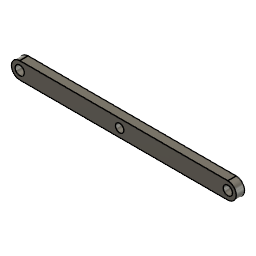
barra_direccion_v3 (Autodesk Fusion 360 design; units mm, degrees)
part number: 2026-03-15-19-52-01-353
Autodesk Fusion 360 part; units mm, degrees
sketch "Boceto1" plane through (0, 0, 0) normal (0, 0, 1) x (1, 0, 0)
  line L0 (0, -23.8223) -> (0, 23.8223) construction
  circle A0 centre (64.256, 0) radius 2.75
  line L1 (-59.344, 5) -> (64.256, 5)
  line L2 (0, 0) -> (11, 0) construction
  line L3 (-59.344, -5) -> (64.256, -5)
  arc A1 (64.256, -5) -> (64.256, 5) centre (64.256, 0) ccw
  circle A2 centre (-59.344, 0) radius 2.75
  arc A3 (-59.344, 5) -> (-59.344, -5) centre (-59.344, 0) ccw
  dimension "d1" = 5.5
  dimension "d2" = 64.256
  dimension "d4" = 10
  dimension "d10" = 5.5
  dimension "d11" = 123.6
  dimension "d12" = 5
  constraint midpoint L0 L2.start
  constraint coincident L2.start origin
  constraint vertical L0
  constraint concentric A0 A1
  constraint tangent L1 A1
  constraint horizontal L1
  constraint perpendicular L0 L2
  constraint symmetric L1.end L2 L3.end
  constraint concentric A2 A3
  constraint tangent L1 A3
  measures "d1" diameter of A0
  measures "d2" distance of L2.start A0.centre
  measures "d4" diameter of A1
  measures "d10" diameter of A2
  measures "d11" distance of A0.centre A2.centre
  measures "d12" distance of L3 A2.centre
extrude "Extruir1" add sketch "Boceto1" along normal blind 5
sketch "Boceto2" plane through (0, 0, 5) normal (0, 0, 1) x (1, 0, 0)
  circle A0 centre (64.256, 0) radius 2.75
  line L0 (-59.344, -5) -> (64.256, -5)
  arc A1 (64.256, -5) -> (64.256, 5) centre (64.256, 0) ccw
  line L1 (64.256, 5) -> (-59.344, 5)
  circle A2 centre (0, 0) radius 2.5
  arc A3 (-59.344, 5) -> (-59.344, -5) centre (-59.344, 0) ccw
  circle A4 centre (-59.344, 0) radius 2.75
  dimension "d8" = 5
  constraint coincident A2.centre origin
  measures "d8" diameter of A2
extrude "Extruir2" cut sketch "Boceto2" against normal through all contours A2
equation "d2 = ( 128.512 / 2 ) * 1 mm"
